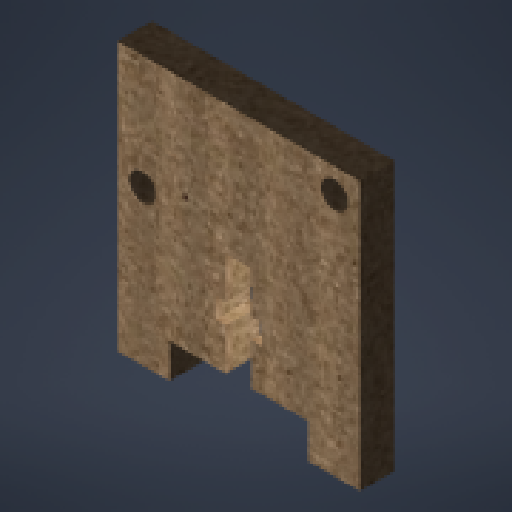
# Autodesk Inventor part: SwitchHolder_V2
Saved by Autodesk Inventor 2024.1 (Build 281209000, 209)
## iProperties
Created: 2022-12-01
Part Number: SwitchHolder_V2
Material: MDF Medium Density Fiberboard
Document SubType Name: Modeling
Designer: jaege
Density: 0.8 g/cm^3
Appearance: Cardboard - Corrugated
Author: jaege
Autodesk Inventor part; units mm, degrees
ref_plane "YZ Plane" through (0, 0, 0) normal (1, 0, 0) x (0, 1, 0)
ref_plane "XZ Plane" through (0, 0, 0) normal (0, 1, 0) x (-1, 0, 0)
ref_plane "XY Plane" through (0, 0, 0) normal (0, 0, 1) x (1, 0, 0)
sketch "Sketch1" plane through (0, 0, 0) normal (0, 0, 1) x (1, 0, 0)
  line L0 (-14, 0) -> (14, 0)
  line L1 (14, 0) -> (14, 16)
  line L2 (14, 16) -> (-14, 16)
  line L3 (-14, 16) -> (-14, 0)
  circle A0 centre (-11.1, 2.85) radius 1.55
  circle A1 centre (11.1, 13.15) radius 1.55
  line L4 (-11.1, 2.85) -> (-14, 2.85) construction
  line L5 (11.1, 13.15) -> (14, 13.15) construction
  line L6 (11.1, 13.15) -> (11.1, 16) construction
  line L7 (-11.1, 2.85) -> (-11.1, 0) construction
  line L8 (-14, 0) -> (14, 0) construction
  line L9 (14, 0) -> (14, -11)
  line L10 (14, -11) -> (8, -11) construction
  line L11 (-14, -11) -> (-14, 0)
  line L12 (-14, -11) -> (-8, -11) construction
  line L13 (-8, -11) -> (-8, -15)
  line L14 (-8, -15) -> (-14, -15)
  line L15 (-14, -15) -> (-14, -11)
  line L16 (14, -11) -> (8, -11) construction
  line L17 (8, -11) -> (8, -15)
  line L18 (8, -15) -> (14, -15)
  line L19 (14, -15) -> (14, -11)
  line L20 (-8, -11) -> (-14, -11) construction
  line L21 (8, -11) -> (-8, -11)
  point P0 (0, 0)
  point P1 (0, 0)
  point P2 (14, 0)
  point P3 (14, 0)
  dimension "d0" = 3.1
  dimension "d1" = 22.2
  dimension "d2" = 10.3
  dimension "d3" = 16
  dimension "d4" = 28
  dimension "d5" = 27
  dimension "d8" = 6
  dimension "d9" = 6
  dimension "d10" = 4
  constraints: 44 end point, 12 parallel, 8 perpendicular, 5 point on line, 4 horizontal, 2 centre point, 1 coincident, 1 collinear, 1 equal radius, 1 horizontal alignment, 1 midpoint
  measures "d0" diameter of A1
  measures "d1" horizontal distance of L5.start L4.start
  measures "d2" vertical distance of L5.start L4.start
  measures "d3" distance of L0.end L1.end
  measures "d4" distance of L1.end L2.end
  measures "d5" distance between parallel lines of L2 L10
  measures "d8" distance of L13.end L14.end
  measures "d9" distance of L18.end L17.end
  measures "d10" distance of L18.end L9.end
extrude "Extrusion1" add sketch "Sketch1" along normal blind 4
sketch "Sketch2" plane through (0, 0, 0) normal (0, 0, -1) x (-1, 0, 0)
  line L0 (8, -11) -> (-8, -11) projected
  line L1 (-1.5, -11) -> (1.5, -11)
  line L2 (1.5, -11) -> (1.5, 1)
  line L3 (1.5, 1) -> (-1.5, 1)
  line L4 (-1.5, 1) -> (-1.5, -11)
  line L5 (-2.7, -6.2) -> (2.7, -6.2)
  line L6 (2.7, -6.2) -> (2.7, -3.8)
  line L7 (2.7, -3.8) -> (-2.7, -3.8)
  line L8 (-2.7, -3.8) -> (-2.7, -6.2)
  point P0 (0, 0)
  point P1 (-2.7, -5)
  point P2 (-1.5, -5)
  point P3 (0, -3.8)
  point P4 (0, 1)
  point P5 (0, -11)
  point P6 (0, -11)
  point P7 (-1.5, -6.2)
  point P8 (1.5, -6.2)
  point P9 (1.5, -3.8)
  point P10 (-1.5, -3.8)
  dimension "d11" = 3
  dimension "d12" = 12
  dimension "d13" = 5.4
  dimension "d14" = 2.4
  constraints: 16 end point, 6 midpoint, 4 parallel, 2 horizontal, 2 perpendicular, 1 coincident, 1 horizontal alignment, 1 point on line, 1 vertical alignment
  measures "d11" distance of L3.end L2.end
  measures "d12" distance of L2.end L1.end
  measures "d13" distance of L7.end L6.end
  measures "d14" distance of L6.end L5.end
extrude "Extrusion2" cut sketch "Sketch2" against normal up to next
body "Solid1"
